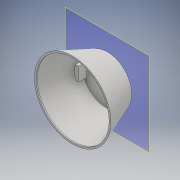
# Autodesk Inventor part: zaklad
Saved by Autodesk Inventor 2017 (Build 210142000, 142)
## iProperties
Created: 2019-02-01
Part Number: zaklad
Material: Generic
Document SubType Name: Modeling
Designer: Denis Kurka
Density: 1 g/cm^3
Appearance: Default
Author: Denis Kurka
Autodesk Inventor part; units mm, degrees
ref_plane "YZ Plane" through (0, 0, 0) normal (1, 0, 0) x (0, 1, 0)
ref_plane "XY Plane" through (0, 0, 0) normal (0, 0, 1) x (1, 0, 0)
sketch "Sketch1" plane through (0, 0, 0) normal (0, 1, 0) x (-1, 0, 0)
  circle A0 centre (0, 0) radius 32
  circle A1 centre (0, 0) radius 33
  dimension "d0" = 64
  dimension "d1" = 0
  dimension "d2" = 0
  dimension "d3" = 66
  constraints: 2 centre point, 1 coincident
  measures "d0" diameter of A0
  measures "d1" distance of point (0, 0) A0.centre
  measures "d2" distance of point (0, 0) A0.centre
  measures "d3" diameter of A1
ref_plane "Work Plane1" through (0, 30, 0) normal (0, 1, 0) x (-1, 0, 0)
sketch "Sketch2" plane through (0, 30, 0) normal (0, 1, 0) x (-1, 0, 0)
  circle A0 centre (0, 0) radius 20
  circle A1 centre (0, 0) radius 21
  dimension "d5" = 40
  dimension "d6" = 42
  constraints: 2 centre point, 2 coincident
  measures "d5" diameter of A0
  measures "d6" diameter of A1
loft "Loft1" add profiles "Sketch2", "Sketch1" contours A0 | A1 / A0 | A1
shell "Shell2" thickness 1 removed faces 0
sketch "Sketch3" plane through (0, 0, 0) normal (0, -1, 0) x (1, 0, 0)
  circle A0 centre (0, 0) radius 31.523
  constraints: 1 centre point, 1 coincident
extrude "Extrusion1" cut sketch "Sketch3" against normal blind 1
sketch "Sketch5" plane through (0, 29, 0) normal (0, -1, 0) x (1, 0, 0)
  line L0 (11.323, 6) -> (6.323, 6)
  line L1 (6.323, 6) -> (6.323, -6)
  line L2 (6.323, -6) -> (11.323, -6)
  line L3 (11.323, -6) -> (11.323, 6)
  circle A0 centre (0, 0) radius 20.323 projected
  circle A1 centre (0, 0) radius 6.323
  circle A2 centre (-6.323, 0) radius 2.5
  line L4 (-16.677, 6) -> (-21.677, 6)
  line L5 (-21.677, 6) -> (-21.677, -6)
  line L6 (-21.677, -6) -> (-16.677, -6)
  line L7 (-16.677, -6) -> (-16.677, 6)
  arc A3 (-19.4171, 6) -> (-19.4171, -6) centre (0, 0) ccw
  dimension "d16" = 5
  dimension "d17" = 12
  dimension "d18" = 9
  dimension "d19" = 6
  dimension "d20" = 5
  dimension "d21" = 5
  dimension "d22" = 12
  dimension "d23" = 23
  constraints: 16 end point, 4 parallel, 4 point on circle, 2 centre point, 2 horizontal, 2 perpendicular, 2 point on line, 1 coincident, 1 concentric, 1 horizontal alignment, 2 other
  measures "d16" distance of L2.end L1.end
  measures "d17" distance of L2.end L0.start
  measures "d18" distance edge to line of A0 L3
  measures "d19" distance from line of point (0, 0) L0
  measures "d20" diameter of A2
  measures "d21" distance of L4.start L4.end
  measures "d22" distance of L4.end L5.end
  measures "d23" distance between parallel lines of L1 L7
extrude "Extrusion2" add sketch "Sketch5" along normal blind 7 contours L3 L2 L1 L0 | A1 A2 | A2 A1 | A1 A2 | L4 L7 L6 A0 picked at (-17.8586, -0.6756)
sketch "Sketch6" plane through (0, 22, 0) normal (0, -1, 0) x (1, 0, 0)
  arc A0 (-5.8287, 2.4507) -> (-5.8287, -2.4507) centre (-6.323, 0) ccw projected
  circle A1 centre (0, 0) radius 6.323
  circle A2 centre (-6.323, 0) radius 2.5
  constraints: 2 coincident, 1 centre point, 1 horizontal alignment, 2 other
extrude "Extrusion3" cut sketch "Sketch6" against normal blind 20
body "Solid1"
